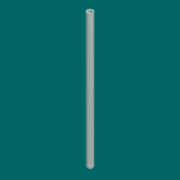
# Autodesk Inventor part: glassTube
Saved by Autodesk Inventor 2016 (Build 200138000, 138)
## iProperties
Created: 2016-09-24
Part Number: glassTube
Material: Glass
Document SubType Name: Modeling
Designer: sawaiz
Density: 2.18 g/cm^3
Appearance: Clear
Author: sawaiz
Autodesk Inventor part; units mm, degrees
ref_plane "YZ Plane" through (0, 0, 0) normal (1, 0, 0) x (0, 1, 0)
ref_plane "XZ Plane" through (0, 0, 0) normal (0, 1, 0) x (-1, 0, 0)
ref_plane "XY Plane" through (0, 0, 0) normal (0, 0, 1) x (1, 0, 0)
sketch "Sketch1" plane through (0, 0, 0) normal (0, 1, 0) x (-1, 0, 0)
  circle A0 centre (0, 0) radius 6.35
  circle A1 centre (0, 0) radius 3.937
  dimension "d0" = 12.7
  dimension "d1" = 7.874
  constraints: 2 centre point, 2 coincident
  measures "d0" diameter of A0
  measures "d1" diameter of A1
extrude "Extrusion1" add sketch "Sketch1" along normal mid plane 273.05
sketch "Sketch2" plane through (0, -136.525, 0) normal (0, -1, 0) x (1, 0, 0)
  circle A0 centre (0, 0) radius 3.937 projected
  circle A1 centre (0, 0) radius 6.35 projected
  circle A2 centre (0, 0) radius 6.35 projected
  line L0 (-6.35, 0) -> (0, 0)
  line L1 (6.35, 0) -> (0, 0)
  circle A3 centre (0, 0) radius 3.937 projected
  arc A4 (3.937, 0) -> (-3.937, 0) centre (0, 0) ccw
  arc A5 (6.35, 0) -> (-6.35, 0) centre (0, 0) ccw
  constraints: 10 point on circle, 4 end point, 2 centre point, 2 horizontal, 2 point on line
revolve "Revolution1" add sketch "Sketch2" angle 180 about axis through (6.35, -136.525, 0) along (1, 0, 0) picked at (-5.446, 0.8206) contours A0 L0 A1 L1
equation "\"d0\" = glassTubeDiameter"
equation "\"d1\" = glassTubeID"
equation "\"d2\" = glassTubeLength - 0.5 * glassTubeDiameter"
equation "\"tubeHeight\" = 50.8"
equation "\"tubeWidth\" = 101.6"
equation "\"tubeLength\" = 304.8"
equation "\"tubeWallThickness\" = 3.175"
equation "\"plateOverhang\" = 6.35"
equation "\"moatWidth\" = 3.175"
equation "\"moatDepth\" = 3.175"
equation "\"tubePlateClearance\" = 0.127"
equation "\"blankCapThickness\" = 9.525"
equation "\"sensorCapThickness\" = 12.7"
equation "\"glassTubeDiameter\" = 12.7"
equation "\"glassTubeClearance\" = 0.19844"
equation "\"glassTubeID\" = 7.874"
equation "\"glassTubeLength\" = 279.4"
equation "\"longHoleSpacing\" = 30.48"
equation "\"shortHoleSpacing\" = 21.59"
equation "\"sensorHolderDiameter\" = 50.8"
equation "\"sensorHolderThickness\" = 12.7"
equation "\"fiberDiameter\" = 1"
equation "\"fiberClearance\" = 0"
equation "\"oRingID\" = 22.2504"
equation "\"oRingGrooveWidth\" = 2.54"
equation "\"oRingGrooveDepth\" = 1.2446"
body "Solid1"
